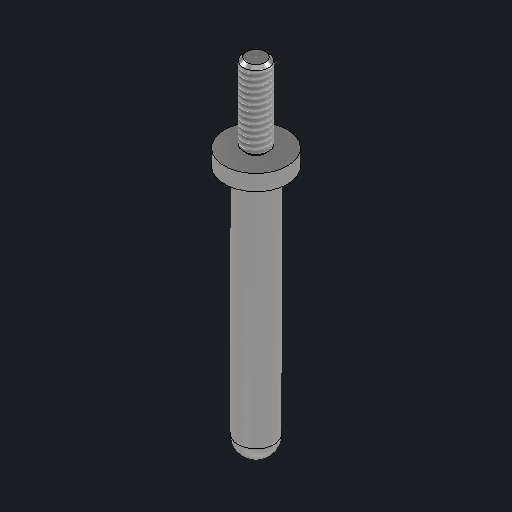
# Autodesk Inventor part: KN-00-03-01
Saved by Autodesk Inventor 2025.2 (Build 292293000, 293)
## iProperties
Created: 2025-04-28
Part Number: KN-00-03-01
Material: X105CrMo17
Document SubType Name: Modeling
Designer: Kacper Mik
Mass: 0.537212 g
Surface Area: 1.01316 cm^2
Volume: 0.0671515 cm^3
Density: 7.75 g/cm^3
Appearance: Semi-Polished
Author: Kacper Mik
Autodesk Inventor part; units mm, degrees
ref_plane "YZ Plane" through (0, 0, 0) normal (1, 0, 0) x (0, 1, 0)
ref_plane "XZ Plane" through (0, 0, 0) normal (0, 1, 0) x (-1, 0, 0)
ref_plane "XY Plane" through (0, 0, 0) normal (0, 0, 1) x (1, 0, 0)
sketch "Sketch1" plane through (0, 0, 0) normal (0, 1, 0) x (-1, 0, 0)
  circle A0 centre (0, 0) radius 2
  dimension "d0" = 4
  constraints: 1 centre point, 1 coincident
  measures "d0" diameter of A0
extrude "Extrusion1" add sketch "Sketch1" against normal blind 1
sketch "Sketch2" plane through (0, 0, 0) normal (0, 1, 0) x (1, 0, 0)
  circle A0 centre (0, 0) radius 0.8
  dimension "d4" = 1.6
  constraints: 1 centre point, 1 coincident
  measures "d4" diameter of A0
extrude "Extrusion2" add sketch "Sketch2" along normal blind 5
thread "Thread1" size "M1.6x0.35" class "6g" standard "ISO Metric profile" full length
sketch "Sketch3" plane through (0, -1, 0) normal (0, -1, 0) x (1, 0, 0)
  circle A0 centre (0, 0) radius 1.15
  dimension "d9" = 2.3
  constraints: 1 centre point, 1 coincident
  measures "d9" diameter of A0
extrude "Extrusion3" add sketch "Sketch3" along normal blind 15.9
fillet "Fillet2" radius 1.15 1 edges at (-1.15, -16.9, 0)
sketch "Sketch4" plane through (0, 0, 0) normal (0, 0, 1) x (1, 0, 0)
  line L0 (-2, -1) -> (2, -1) projected
  line L1 (2, 0) -> (-2, 0) projected
  line L2 (0.8, 5) -> (-0.8, 5) projected
  line L3 (-0.8, 0) -> (0.8, 0) projected
  line L4 (0.8, 0) -> (0.6, 0)
  line L5 (0.6, 0) -> (0.6, 0.2)
  line L6 (0.6, 0.2) -> (0.8, 0.2)
  line L7 (0.8, 0.2) -> (0.8, 0)
  line L8 (0, -2.2) -> (0, 6.2) projected
  point P0 (0, 0)
  dimension "d13" = 0.2
  dimension "d14" = 0.2
  constraints: 8 end point, 2 parallel, 1 horizontal, 1 perpendicular
  measures "d13" distance of L5.end L6.end
  measures "d14" distance of L4.end L5.end
revolve "Revolution1" cut sketch "Sketch4" angle 360 about axis through (0, -10, 0) along (0, 1, 0)
chamfer "Chamfer1" distance 0.2 angle 45 1 edges at (-0.8, 5, 0)
equation "\"d12\" = 0.5 * d9"
body "Solid1"
